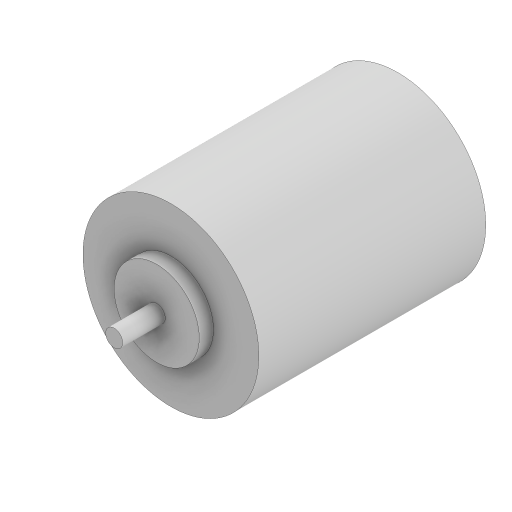
# Autodesk Inventor part: MOTOR DC
Saved by Autodesk Inventor 2024 (Build 280153000, 153)
## iProperties
Created: 2024-05-26
Part Number: MOTOR DC
Material: Generic
Document SubType Name: Modeling
Designer: Jhuliams
Density: 1 g/cm^3
Appearance: Default
Author: Jhuliams
Autodesk Inventor part; units mm, degrees
ref_plane "YZ Plane" through (0, 0, 0) normal (1, 0, 0) x (0, 1, 0)
ref_plane "XZ Plane" through (0, 0, 0) normal (0, 1, 0) x (-1, 0, 0)
ref_plane "XY Plane" through (0, 0, 0) normal (0, 0, 1) x (1, 0, 0)
sketch "Sketch1" plane through (0, 0, 0) normal (0, 0, 1) x (1, 0, 0)
  circle A0 centre (0, 0) radius 31
  dimension "d0" = 62
  constraints: 1 centre point, 1 coincident
  measures "d0" diameter of A0
extrude "Extrusion1" add sketch "Sketch1" along normal mid plane 80
sketch "Sketch2" plane through (0, 0, 40) normal (0, 0, 1) x (1, 0, 0)
  circle A0 centre (0, 0) radius 3
  dimension "d3" = 6
  constraints: 1 centre point, 1 coincident
  measures "d3" diameter of A0
extrude "Extrusion2" add sketch "Sketch2" along normal blind 20
sketch "Sketch3" plane through (0, 0, 40) normal (0, 0, 1) x (1, 0, 0)
  circle A0 centre (0, 0) radius 3 projected
  circle A1 centre (0, 0) radius 15
  dimension "d6" = 30
  constraints: 1 centre point, 1 coincident
  measures "d6" diameter of A1
extrude "Extrusion3" add sketch "Sketch3" along normal blind 5
body "Solid1"
